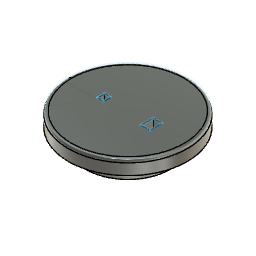
Turbidity Sensor End Cap F3D File (Autodesk Fusion 360 design; units mm, degrees)
Autodesk Fusion 360 part; units mm, degrees
sketch "Sketch1" plane through (0, 0, 0) normal (0, 0, 1) x (1, 0, 0)
  circle A0 centre (0, 0) radius 38.1
  dimension "d1" = 76.2
  constraint coincident A0.centre origin
  measures "d1" diameter of A0
extrude "Extrude1" add sketch "Sketch1" along normal blind 19.05
sketch "Sketch2" plane through (0, 0, 19.05) normal (0, 0, 1) x (-1, 0, 0)
  circle A0 centre (0, 0) radius 38.1
  line L0 (17, -2) -> (13.15, -2)
  line L1 (13.15, -2) -> (13.15, 2.5)
  line L2 (13.15, 2.5) -> (17, 2.5)
  line L3 (17, 2.5) -> (17, -2)
  line L4 (-12.23, -4) -> (-18, -4)
  line L5 (-18, -4) -> (-18, 3.8)
  line L6 (-18, 3.8) -> (-12.23, 3.8)
  line L7 (-12.23, 3.8) -> (-12.23, -4)
  dimension "d4" = 4.5
  dimension "d5" = 3.85
  dimension "d6" = 5.77
  dimension "d7" = 7.8
  constraint horizontal L0
  constraint vertical L1
  constraint horizontal L2
  constraint vertical L3
  constraint horizontal L4
  constraint vertical L5
  constraint horizontal L6
  constraint vertical L7
  measures "d4" distance of L0.start L2.end
  measures "d5" distance of L1 L3
  measures "d6" distance of L5 L7
  measures "d7" distance of L4 L6
extrude "Extrude2" cut sketch "Sketch2" against normal blind 8.8 contours L4 L5 L6 L7
sketch "Sketch3" plane through (0, 0, 19.05) normal (0, 0, 1) x (-1, 0, 0)
  line L0 (-18, -4) -> (-18, 3.8)
  line L1 (-18, 3.8) -> (-12.23, 3.8)
  line L2 (-12.23, 3.8) -> (-12.23, -4)
  line L3 (-12.23, -4) -> (-18, -4)
  circle A0 centre (0, 0) radius 38.1
  line L4 (16.845, -2) -> (13, -2)
  line L5 (13, -2) -> (13, 2.5)
  line L6 (13, 2.5) -> (16.845, 2.5)
  line L7 (16.845, 2.5) -> (16.845, -2)
  dimension "d10" = 3.845
  dimension "d11" = 4.5
  constraint horizontal L4
  constraint vertical L5
  constraint horizontal L6
  constraint vertical L7
  measures "d10" distance of L5 L7
  measures "d11" distance of L4 L6
extrude "Extrude3" cut sketch "Sketch3" against normal blind 3.75 contours L4 L5 L6 L7
sketch "Sketch4" plane through (0, 0, 19.05) normal (0, 0, 1) x (1, 0, 0)
sketch "Sketch5" plane through (0, 0, 0) normal (0, 0, 1) x (1, 0, 0)
  circle A0 centre (-15, 0) radius 1.4142
extrude "Extrude4" cut sketch "Sketch5" along normal blind 21
sketch "Sketch6" plane through (0, 0, 0) normal (0, 0, 1) x (1, 0, 0)
  circle A0 centre (15, 0) radius 1.4142
extrude "Extrude5" cut sketch "Sketch6" along normal blind 19
sketch "Sketch7" plane through (0, 0, 19.05) normal (0, 0, 1) x (1, 0, 0)
fillet "Fillet1" radius 2 tangency weight 2 1 edges at (-35.5217, -13.7775, 19.05)
torus "TorusPrimitive1" cut centre line diameter 74.095 section diameter 20 placed x (1, 0, 0) y (0, 1, 0) z (0, 0, 1) at (0, 0, 0)
